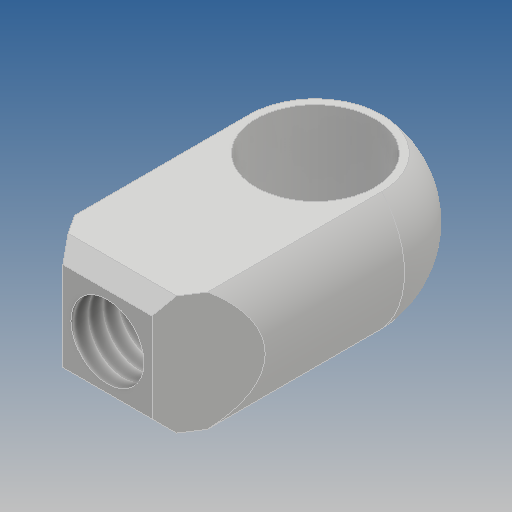
# Autodesk Inventor part: Pleuelkopf
Saved by Autodesk Inventor 2018 (Build 220112000, 112)
## iProperties
Created: 2018-10-09
Part Number: Pleuelkopf
Material: Generisch
Document SubType Name: Modeling
Designer: M.Knabel
Density: 1 g/cm^3
Appearance: Vorgabe
Mass: 0.121409 g
Surface Area: 2.44027 cm^2
Volume: 0.121409 cm^3
Author: M.Knabel
Autodesk Inventor part; units mm, degrees
ref_plane "YZ Plane" through (0, 0, 0) normal (1, 0, 0) x (0, 1, 0)
ref_plane "XZ Plane" through (0, 0, 0) normal (0, 1, 0) x (-1, 0, 0)
ref_plane "XY Plane" through (0, 0, 0) normal (0, 0, 1) x (1, 0, 0)
sketch "Skizze1" plane through (0, 0, 0) normal (0, 0, 1) x (1, 0, 0)
  line L0 (-1.2, 0) -> (7.2, 0) projected
  line L1 (0, -2) -> (0, 12) projected
  line L2 (0, 7) -> (0, 2.3098)
  line L3 (0, 2.3098) -> (1.5, 0)
  line L4 (1.5, 0) -> (4.5, 0)
  line L5 (4.5, 0) -> (6, 2.3098)
  line L6 (6, 2.3098) -> (6, 7)
  arc A0 (6, 7) -> (0, 7) centre (3, 7) ccw
  point P0 (0, 0)
  dimension "d0" = 33
  dimension "d1" = 33
  dimension "d2" = 3
  dimension "d3" = 10
  dimension "d4" = 1.5
  dimension "d5" = 3
  constraints: 10 end point, 4 point on line, 2 point on circle, 2 tangent, 1 centre point, 1 parallel
  measures "d0" angle of L3 L1
  measures "d1" angle of L6 L5
  measures "d2" radius of A0
  measures "d4" distance from line of L3.end L1
  measures "d5" distance of L4.end L3.end
extrude "Extrusion1" add sketch "Skizze1" along normal mid plane 4 contours L3 L1 A0 L6 L5 L0
sketch "Skizze2" plane through (0, 0, -2) normal (0, 0, -1) x (-1, 0, 0)
  arc A0 (0, 7) -> (-6, 7) centre (-3, 7) ccw projected
  point P0 (0, 0)
  constraints: 1 coincident
hole "Bohrung1" at (3, 7, -2) at (3, 7, -2) direction (0, 0, 1) diameter 4 end through all
sketch "Skizze3" plane through (1.5, 0, 2) normal (0, -1, 0) x (1, 0, 0)
  line L0 (-2.7, -2) -> (5.7, -2) projected
  line L1 (-1.5, -4.8) -> (-1.5, 0.8) projected
  point P0 (-1.5, -2)
  point P1 (1.5, -2)
  dimension "d15" = 3
  constraints: 1 midpoint
  measures "d15" distance from line of point (1.5, -2) L1
hole "Bohrung2" at (3, 0, 0) direction (0, 1, 0) diameter 2.459 depth 4 tip angle 118
sketch "Skizze4" plane through (1.5, 0, 2) normal (0, -1, 0) x (1, 0, 0)
  arc A0 (3.7361, -4) -> (3.7361, 0) centre (1.5, -2) ccw
  line L0 (3.7361, 0) -> (5.5, 0)
  line L1 (5.5, 0) -> (5.5, -4)
  line L2 (5.5, -4) -> (3.7361, -4)
  line L3 (4.5, -4) -> (3, -4) projected
  line L4 (3, 0) -> (4.5, 0) projected
  line L5 (4.5, -4) -> (4.5, 0) projected
  dimension "d24" = 3
  dimension "d25" = 4
  constraints: 6 end point, 2 collinear, 2 point on circle, 1 centre point, 1 coincident, 1 horizontal, 1 perpendicular
  measures "d24" radius of A0
  measures "d25" distance from line of point (1.5, -2) L1
sketch "Skizze5" plane through (0, 0, 2) normal (0, 0, 1) x (1, 0, 0)
  line L0 (6, 0) -> (6, 7)
  line L1 (6, 2.3098) -> (6, 7) projected
  arc A0 (6, 7) -> (0, 7) centre (3, 7) ccw projected
  line L2 (0, 7) -> (0, 2.3098) projected
  arc A1 (6, 7) -> (0, 7) centre (3, 7) ccw
  line L3 (0, 7) -> (0, 0)
  constraints: 5 end point, 2 point on circle, 2 vertical, 1 centre point, 1 coincident, 1 collinear, 1 concentric
sweep "Sweeping2" cut profiles "Skizze4" path "Skizze5" path curves L0 A1 L3
chamfer "Fase2" distance 0.5 angle 45 2 edges at (3, 0, 2) (3, 0, -2)
